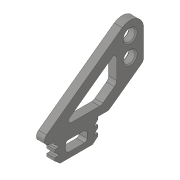
# Autodesk Inventor part: M2_LINKAGE
Saved by Autodesk Inventor 2019 (Build 230136000, 136)
## iProperties
Created: 2022-04-02
Part Number: M2_LINKAGE
Material: ABS Plastic
Document SubType Name: Modeling
Designer: solyo
Density: 1.06 g/cm^3
Appearance: Smooth - Medium Gray
Mass: 0.17676 g
Surface Area: 3.85692 cm^2
Volume: 0.166755 cm^3
Author: solyo
Autodesk Inventor part; units mm, degrees
ref_plane "YZ Plane" through (0, 0, 0) normal (1, 0, 0) x (0, 1, 0)
ref_plane "XZ Plane" through (0, 0, 0) normal (0, 1, 0) x (-1, 0, 0)
sketch "Sketch1" plane through (0, 0, 0) normal (1, 0, 0) x (0, 1, 0)
  line L0 (0, 0) -> (12.0218, -16.5295)
  line L1 (10, -20.5) -> (4.7274, -20.5)
  line L2 (0, -14) -> (4.7274, -20.5)
  line L3 (0, 0) -> (0, -4)
  line L4 (0, -4) -> (-4, -4)
  line L5 (-4, -4) -> (-4, -12)
  line L6 (-4, -12) -> (0, -12)
  line L7 (0, -12) -> (0, -14)
  arc A0 (10, -20.5) -> (12.0218, -16.5295) centre (10, -18) ccw
  point P0 (14.9095, -20.5)
  point P1 (6.5, -18)
  dimension "d26" = 8
  dimension "d31" = 4
  dimension "d32" = 2
  dimension "d43" = 2.5
  dimension "d45" = 10
  dimension "d64" = 3.5
  dimension "d65" = 4
  dimension "d78" = 18
  constraints: 16 end point, 3 parallel, 3 point on line, 2 horizontal, 2 point on circle, 2 tangent, 1 centre point, 1 coincident, 1 collinear, 1 vertical
  measures "d26" distance of L4.end L5.end
  measures "d31" distance between parallel lines of L3 L5
  measures "d32" distance of L6.end L2.start
  measures "d43" radius of A0
  measures "d45" horizontal distance of L0.start point (10, -18)
  measures "d64" distance of A0.centre point (6.5, -18)
  measures "d65" distance of L0.start L3.end
  measures "d78" vertical distance of L0.start point (10, -18)
extrude "Extrusion1" add sketch "Sketch1" along normal blind 1.5
hole "Hole3" at (0, 10, -18) at (0, 6.5, -18) direction (1, 0, 0) diameter 2.2 end through all
fillet "Fillet3" radius 1 3 edges at (0.75, 0, 0) (0.75, 4.7274, -20.5) (0.75, 0, -14)
chamfer "Chamfer2" distance 0.2 angle 45 4 edges at (1.5, 6.5, -19.1) (1.5, 10, -19.1) (0, 6.5, -19.1) (0, 10, -19.1)
ref_plane "Work Plane1" through (0, -4, -8) normal (0, 0, -1) x (-1, 0, 0)
sketch "Sketch4" plane through (1.5, 0, 0) normal (1, 0, 0) x (0, 0, -1)
  arc A0 (2.4869, 1.8087) -> (3.0751, 0) centre (3.0751, 1) ccw projected
  line L0 (3.0751, 0) -> (4, 0) projected
  line L1 (4, 0) -> (4, -4) projected
  line L2 (4, -4) -> (12, -4) projected
  line L3 (12, -4) -> (12, 0) projected
  line L4 (12, 0) -> (13.6748, 0) projected
  line L5 (14.263, 0.1913) -> (20.0882, 4.4279) projected
  line L6 (20.5, 5.2366) -> (20.5, 10) projected
  arc A1 (20.5, 10) -> (16.5295, 12.0218) centre (18, 10) ccw projected
  line L7 (16.5295, 12.0218) -> (2.4869, 1.8087) projected
  circle A2 centre (18, 10) radius 1.3 projected
  line L8 (4, 0) -> (12, 0)
  line L9 (12, -4) -> (4, -4) projected
  line L10 (5, -4) -> (4, -3.1667)
  line L11 (4, -4) -> (4, 0) projected
  line L12 (4, -2.6667) -> (5, -2.6667)
  line L13 (5, -2.6667) -> (4, -1.8333)
  line L14 (4, -1.3333) -> (5, -1.3333)
  line L15 (5, -1.3333) -> (4, -0.5)
  line L16 (4, -0.5) -> (4, 0)
  line L17 (4, -0.5) -> (4, -1.3333)
  line L18 (4, -1.8333) -> (4, -2.6667)
  line L19 (4, -3.1667) -> (4, -4)
  line L20 (4, -4) -> (5, -4)
  arc A3 (13.6748, 0) -> (14.263, 0.1913) centre (13.6748, 1) ccw projected
  arc A4 (20.0882, 4.4279) -> (20.5, 5.2366) centre (19.5, 5.2366) ccw projected
  point P0 (0, 0)
  dimension "d57" = 1
  dimension "d58" = 0.5
  dimension "d59" = 0.5
  dimension "d60" = 0.5
  constraints: 22 end point, 6 point on line, 3 collinear, 3 perpendicular, 2 parallel, 2 vertical alignment, 1 horizontal, 1 vertical
  measures "d57" distance of L1.end L10.start
  measures "d58" distance of L13.end L14.start
  measures "d59" distance of L12.start L10.end
  measures "d60" distance of L15.end L0.end
extrude "Extrusion2" cut sketch "Sketch4" against normal through all contours L15 L14 L1 | L13 L12 L1 | L2 L1 L10
mirror "Mirror1" about plane through (0, -4, -8) normal (0, 0, -1) of "Extrusion2"
fillet "Fillet4" radius 0.2 4 edges at (0.75, -1.3333, -11) (0.75, -2.6667, -11) (0.75, -1.3333, -5) (0.75, -2.6667, -5)
sketch "Sketch5" plane through (1.5, 0, 0) normal (1, 0, 0) x (0, 0, -1)
  line L0 (5.4627, 1.5) -> (12.6621, 1.5)
  line L1 (12.6621, 1.5) -> (15.5, 3.564)
  line L2 (15.5, 3.564) -> (15.5, 8.8)
  line L3 (15.5, 8.8) -> (5.4627, 1.5)
  line L4 (16.5295, 12.0218) -> (2.4869, 1.8087) projected
  circle A0 centre (18, 6.5) radius 1.3 projected
  line L5 (14.263, 0.1913) -> (20.0882, 4.4279) projected
  line L6 (12, 0) -> (13.6748, 0) projected
  line L7 (6, -1) -> (10, -1)
  line L8 (10, -1) -> (10, -3)
  line L9 (10, -3) -> (6, -3)
  line L10 (6, -3) -> (6, -1)
  line L11 (5, -4) -> (11, -4) projected
  line L12 (12, -0.5) -> (12, 0) projected
  line L13 (4, 0) -> (4, -0.5) projected
  point P0 (0, 0)
  point P1 (14, 0)
  point P2 (21.5, 5.144)
  dimension "d66" = 2.5
  dimension "d67" = 2
  dimension "d68" = 2
  dimension "d69" = 1.5
  dimension "d74" = 1
  dimension "d75" = 1
  dimension "d76" = 2
  dimension "d77" = 2
  constraints: 16 end point, 4 parallel, 2 horizontal, 1 perpendicular, 1 vertical, 1 other
  measures "d66" distance from line of L2 A0.centre
  measures "d67" distance between parallel lines of L4 L3
  measures "d69" distance between parallel lines of L6 L0
  measures "d74" distance between parallel lines of L11 L9
  measures "d75" distance between parallel lines of L6 L7
  measures "d76" distance between parallel lines of L12 L8
  measures "d77" distance between parallel lines of L13 L10
extrude "Extrusion3" cut sketch "Sketch5" against normal through all contours L3 L2 L1 L0 | L7 L8 L9 L10
fillet "Fillet5" radius 0.5 6 edges at (0.75, 1.5, -5.4627) (0.75, 8.8, -15.5) (0.75, -3, -6) (0.75, -1, -6) (0.75, -1, -10) (0.75, -3, -10)
fillet "Fillet5" radius 1 2 edges at (0.75, 3.564, -15.5) (0.75, 1.5, -12.6621)
equation "\"d46\" = hole_diameter"
equation "\"d59\" = d58"
equation "\"d60\" = d58"
equation "\"d68\" = d67"
equation "\"d77\" = d76"
equation "\"d1\" = d0"
equation "\"d21\" = d1"
equation "\"hole_diameter\" = 2.2"
equation "\"d0\" = 12"
body "Solid1"
